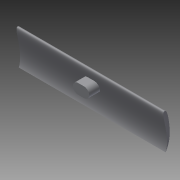
# Autodesk Inventor part: 2015 Back Spoiler 1
Saved by Autodesk Inventor 2015 (Build 190159000, 159)
## iProperties
Created: 2015-03-25
Part Number: 2015 Back Spoiler 1
Material: Generic
Document SubType Name: Modeling
Designer: Lks112201918
Density: 1 g/cm^3
Appearance: Default
Author: Lks112201918
Autodesk Inventor part; units mm, degrees
ref_plane "YZ Plane" through (0, 0, 0) normal (1, 0, 0) x (0, 1, 0)
ref_plane "XZ Plane" through (0, 0, 0) normal (0, 1, 0) x (-1, 0, 0)
ref_plane "XY Plane" through (0, 0, 0) normal (0, 0, 1) x (1, 0, 0)
sketch "Sketch1" plane through (0, 0, 0) normal (1, 0, 0) x (0, 1, 0)
  line L0 (0, 0) -> (10, 0)
  line L1 (10, 0) -> (10, -18)
  line L2 (10, -18) -> (0, -18)
  line L3 (0, -18) -> (0, 0)
  spline S0 degree 4 poles (3.4811, -17.7286) (4.0754, -16.5984) (6.7935, -13.1301) (4.9927, -3.6489) (3.9933, 0.2842) (2.722, 0) knots 0 0 0 0 0 0.526556 1 1 1 1 1
  spline S1 degree 3 poles (2.722, 0) (1.0371, -0.5817) (5.854, -12.0092) (3.4811, -17.7286) knots 0 0 0 0 1 1 1 1
  point P0 (4.392, -16.0283)
  point P1 (5.4548, -11.4431)
  point P2 (4.8476, -3.8821)
  point P3 (3.6937, -0.39)
  point P4 (2.3577, -0.8758)
  point P5 (3.4812, -7.5865)
  dimension "d0" = 10
  dimension "d1" = 18
  constraints: 8 end point, 2 parallel, 1 horizontal, 1 perpendicular, 1 point on line, 10 other
  measures "d0" distance of L1.end L2.end
  measures "d1" distance of L0.end L1.end
extrude "Extrusion1" add sketch "Sketch1" along normal blind 36 contours S0 L0 | L0 S0 S1
sketch "Sketch2" plane through (36, 0, 0) normal (1, 0, 0) x (0, 0, -1)
  line L0 (4.2519, 4) -> (9.2519, 4)
  line L1 (9.2519, 4) -> (9.2519, 0)
  line L2 (9.2519, 0) -> (4.2519, 0)
  line L3 (4.2519, 0) -> (4.2519, 4)
  point P0 (0, 0)
  dimension "d4" = 5
  dimension "d7" = 4
  constraints: 8 end point, 2 parallel, 1 horizontal, 1 perpendicular
  measures "d4" distance of L1.end L2.end
  measures "d7" distance of L2.end L0.start
extrude "Extrusion2" add sketch "Sketch2" against normal blind 4
mirror "Mirror1" about plane through (36, 4.1406, -8.6966) normal (1, 0, 0)
sketch "Sketch3" plane through (32, 0, -9.2519) normal (0, -1, 0) x (1, 0, 0)
  line L0 (0, 5) -> (8, 5)
  line L1 (8, 5) -> (8, 0)
  line L2 (8, 0) -> (0, 0)
  line L3 (0, 0) -> (0, 5)
  point P0 (-32, 9.2519)
  constraints: 8 end point, 2 parallel, 1 horizontal, 1 perpendicular
extrude "Extrusion3" add sketch "Sketch3" along normal blind 2
fillet "Fillet1" radius 2.5 1 edges at (40, 0.4133, -4.2519)
fillet "Fillet2" radius 2.5 1 edges at (32, 0.4133, -4.2519)
fillet "Fillet3" radius 2.5 1 edges at (40, 0.8821, -9.2519)
fillet "Fillet4" radius 2.5 1 edges at (32, 0.8821, -9.2519)
body "Solid1"
